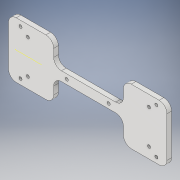
# Autodesk Inventor part: top plate
Saved by Autodesk Inventor 2019 (Build 230136000, 136)
## iProperties
Created: 2019-10-06
Part Number: top plate
Material: UHMW, White
Document SubType Name: Modeling
Designer: robgr
Density: 0.94 g/cm^3
Appearance: Smooth - White
Mass: 34.1715 g
Surface Area: 211.61 cm^2
Volume: 36.3527 cm^3
Author: robgr
Autodesk Inventor part; units mm, degrees
ref_plane "YZ Plane" through (0, 0, 0) normal (1, 0, 0) x (0, 1, 0)
sketch "Sketch1" plane through (0, 0, 0) normal (0, 0, 1) x (1, 0, 0)
  line L0 (-19.3782, 63.0791) -> (164.6218, 63.0791)
  line L1 (174.6218, 53.0791) -> (174.6218, 1.0791)
  line L2 (164.6218, -8.9209) -> (-19.3782, -8.9209)
  line L3 (-29.3782, 1.0791) -> (-29.3782, 53.0791)
  arc A0 (-19.3782, 63.0791) -> (-29.3782, 53.0791) centre (-19.3782, 53.0791) ccw
  arc A1 (-29.3782, 1.0791) -> (-19.3782, -8.9209) centre (-19.3782, 1.0791) ccw
  arc A2 (164.6218, -8.9209) -> (174.6218, 1.0791) centre (164.6218, 1.0791) ccw
  arc A3 (174.6218, 53.0791) -> (164.6218, 63.0791) centre (164.6218, 53.0791) ccw
  point P0 (0, 0)
  point P1 (-29.3782, 63.0791)
  point P2 (174.6218, -8.9209)
  point P3 (-29.3782, -8.9209)
  dimension "d0" = 204
  dimension "d1" = 72
  dimension "d2" = 10
  constraints: 8 end point, 8 point on circle, 8 tangent, 6 point on line, 4 centre point, 3 equal radius, 2 parallel, 1 horizontal, 1 perpendicular
  measures "d0" distance of point (174.622, -8.921) point (-29.378, -8.921)
  measures "d1" distance of point (-29.378, -8.921) point (-29.378, 63.079)
  measures "d2" radius of A0
extrude "Extrusion1" add sketch "Sketch1" along normal blind 6
sketch "Sketch4" plane through (0, 0, 6) normal (0, 0, 1) x (1, 0, 0)
  circle A0 centre (-4.3782, 5.0791) radius 2
  circle A1 centre (-19.3782, 14.5791) radius 2 projected
  circle A2 centre (-4.3782, 49.0791) radius 2
  circle A3 centre (-19.3782, 39.5791) radius 2 projected
  line L0 (164.6218, 63.0791) -> (-19.3782, 63.0791) projected
  line L1 (72.6218, 63.0791) -> (72.6218, -8.9209)
  line L2 (-19.3782, -8.9209) -> (164.6218, -8.9209) projected
  circle A4 centre (151.6218, 5.0791) radius 2
  circle A5 centre (151.6218, 49.0791) radius 2
  line L3 (-29.3782, 53.0791) -> (-29.3782, 1.0791) projected
  point P0 (0, 0)
  dimension "d17" = 4
  dimension "d19" = 4
  dimension "d38" = 14
  dimension "d39" = 14
  dimension "d40" = 25
  dimension "d41" = 25
  dimension "d43" = 156
  dimension "d44" = 156
  dimension "d45" = 79
  constraints: 4 centre point, 2 end point, 2 midpoint
  measures "d17" diameter of A0
  measures "d19" diameter of A2
  measures "d38" distance from line of L0 A2.centre
  measures "d39" distance from line of A0.centre L2
  measures "d40" distance from line of L3 A0.centre
  measures "d41" distance from line of L3 A2.centre
  measures "d43" distance of A2.centre A5.centre
  measures "d44" distance of A0.centre A4.centre
  measures "d45" distance from line of L1 A4.centre
extrude "Extrusion4" cut sketch "Sketch4" against normal blind 6 contours A0 | A2 | A4 | A5
ref_plane "Work Plane1" through (74.6218, 1.0791, 0) normal (1, 0, 0) x (0, 0, -1)
ref_plane "Work Plane2" through (-19.3782, 27.0791, 0) normal (0, -1, 0) x (1, 0, 0)
sketch "Sketch5" plane through (0, 0, 0) normal (0, 0, -1) x (-1, 0, 0)
  line L0 (-41.6218, -8.9209) -> (-72.6218, -8.9209)
  line L1 (-72.6218, -8.9209) -> (-72.6218, 21.0791)
  line L2 (-72.6218, 21.0791) -> (-41.6218, 21.0791)
  line L3 (-41.6218, 21.0791) -> (-41.6218, -8.9209)
  line L4 (19.3782, -8.9209) -> (-164.6218, -8.9209) projected
  line L5 (-164.6218, 63.0791) -> (19.3782, 63.0791) projected
  line L6 (-72.6218, -8.9209) -> (-103.6218, -8.9209)
  line L7 (-103.6218, -8.9209) -> (-103.6218, 21.0791)
  line L8 (-103.6218, 21.0791) -> (-72.6218, 21.0791)
  line L9 (-72.6218, 21.0791) -> (-72.6218, -8.9209)
  line L10 (-43.8163, 63.0791) -> (-72.6218, 63.0791)
  line L11 (-72.6218, 63.0791) -> (-72.6218, 33.0791)
  line L12 (-72.6218, 33.0791) -> (-53.8163, 33.0791)
  line L13 (-43.8163, 32.0791) -> (-43.8163, 63.0791)
  line L14 (-72.6218, 33.0791) -> (-93.6218, 33.0791)
  line L15 (-103.6218, 31.0791) -> (-103.6218, 63.0791)
  line L16 (-103.6218, 63.0791) -> (-72.6218, 63.0791)
  line L17 (-72.6218, 63.0791) -> (-72.6218, 33.0791)
  line L18 (-41.6218, -8.9209) -> (-6.6218, -8.9209)
  line L19 (-43.8163, 63.0791) -> (-11.7113, 63.0791)
  line L20 (-103.6218, -8.9209) -> (-138.6218, -8.9209)
  line L21 (-103.6218, 63.0791) -> (-138.6218, 63.0791)
  line L22 (-43.8163, 63.0791) -> (-28.8163, 63.0791)
  line L23 (-28.8163, 63.0791) -> (-28.8163, 51.444)
  line L24 (-43.8163, 32.0791) -> (-43.8163, 63.0791)
  line L25 (-103.6218, 63.0791) -> (-118.6218, 63.0791)
  line L26 (-118.6218, 63.0791) -> (-118.6218, 50.444)
  line L27 (-103.6218, 31.0791) -> (-103.6218, 63.0791)
  line L28 (-72.6218, -8.9209) -> (-72.6218, 21.0791)
  line L29 (-72.6218, 33.0791) -> (-72.6218, 63.0791)
  line L30 (-28.8163, 51.444) -> (-28.8163, 43.0791)
  line L31 (-38.8163, 33.0791) -> (-53.8163, 33.0791)
  line L32 (-93.6218, 33.0791) -> (-108.6218, 33.0791)
  line L33 (-118.6218, 43.0791) -> (-118.6218, 50.444)
  arc A0 (-38.8163, 33.0791) -> (-28.8163, 43.0791) centre (-38.8163, 43.0791) ccw
  arc A1 (-118.6218, 43.0791) -> (-108.6218, 33.0791) centre (-108.6218, 43.0791) ccw
  line L34 (29.3782, 1.0791) -> (29.3782, 53.0791) projected
  point P0 (0, 0)
  dimension "d25" = 31
  dimension "d26" = 30
  dimension "d27" = 31
  dimension "d28" = 30
  dimension "d29" = 35
  dimension "d30" = 35
  dimension "d46" = 15
  dimension "d47" = 15
  dimension "d48" = 10
  dimension "d61" = 102
  constraints: 64 end point, 10 parallel, 8 point on line, 7 horizontal, 6 perpendicular, 4 point on circle, 4 tangent, 2 centre point, 2 midpoint, 2 vertical, 1 equal radius
  measures "d25" distance of L0.end L0.start
  measures "d26" distance of L0.end L1.end
  measures "d27" distance of L7.end L1.end
  measures "d28" distance of L11.end L10.end
  measures "d29" distance of L0.start L18.end
  measures "d30" distance of L6.end L20.end
  measures "d46" distance between parallel lines of L13 L23
  measures "d47" distance between parallel lines of L15 L26
  measures "d48" radius of A0
  measures "d61" distance between parallel lines of L34 L17
extrude "Extrusion5" cut sketch "Sketch5" against normal blind 6 contours L5 L15 L32 A1 L33 L26 | L5 L11 L14 L32 L15 | L5 L13 L31 L12 L11 | L5 L23 L30 A0 L31 L13
ref_plane "Work Plane3" through (-19.3782, 27.0791, 6) normal (0, 1, 0) x (1, 0, 0)
mirror "Mirror1" about plane through (-19.3782, 27.0791, 6) normal (0, 1, 0) of "Extrusion5"
fillet "Fillet1" radius 10 4 edges at (118.6218, 63.0791, 3) (28.8163, 63.0791, 3) (28.8163, -8.9209, 3) (118.6218, -8.9209, 3)
sketch "Sketch7" plane through (0, 0, 0) normal (0, 0, -1) x (-1, 0, 0)
  circle A0 centre (13.8782, -1.9209) radius 2
  circle A1 centre (13.8782, 56.0791) radius 2
  circle A2 centre (-161.1218, 56.0791) radius 2
  circle A3 centre (-161.1218, -1.9209) radius 2
  line L0 (-28.8163, 53.0791) -> (-28.8163, 43.0791) projected
  line L1 (-28.8163, 11.0791) -> (-28.8163, 1.0791) projected
  line L2 (-118.6218, 1.0791) -> (-118.6218, 11.0791) projected
  line L3 (-118.6218, 43.0791) -> (-118.6218, 53.0791) projected
  point P0 (0, 0)
  point P1 (-161.1218, 5.0791)
  dimension "d49" = 4
  dimension "d50" = 4
  dimension "d54" = 7
  dimension "d57" = 42.6945
  dimension "d58" = 42.6945
  dimension "d59" = 42.5
  dimension "d60" = 42.5
  constraints: 4 centre point
  measures "d49" diameter of A0
  measures "d50" diameter of A1
  measures "d54" distance of point (-161.122, 5.079) A3.centre
  measures "d57" distance from line of L0 A1.centre
  measures "d58" distance from line of L1 A0.centre
  measures "d59" distance from line of A3.centre L2
  measures "d60" distance from line of L3 A2.centre
extrude "Extrusion6" cut sketch "Sketch7" against normal blind 6
sketch "Sketch8" plane through (0, 0, 6) normal (0, 0, 1) x (1, 0, 0)
  line L0 (-29.3782, 1.0791) -> (-29.3782, 53.0791) projected
  line L1 (-29.3782, 27.0791) -> (174.6218, 27.0791)
  line L2 (174.6218, 53.0791) -> (174.6218, 1.0791) projected
  circle A0 centre (45.6218, 27.0791) radius 2
  circle A1 centre (99.6218, 27.0791) radius 2
  point P0 (0, 0)
  dimension "d62" = 4
  dimension "d63" = 4
  dimension "d64" = 75
  dimension "d65" = 75
  constraints: 2 centre point, 2 end point, 2 midpoint, 2 point on line
  measures "d62" diameter of A0
  measures "d63" diameter of A1
  measures "d64" distance from line of L0 A0.centre
  measures "d65" distance from line of L2 A1.centre
extrude "Extrusion7" cut sketch "Sketch8" against normal blind 6
body "Solid1"
